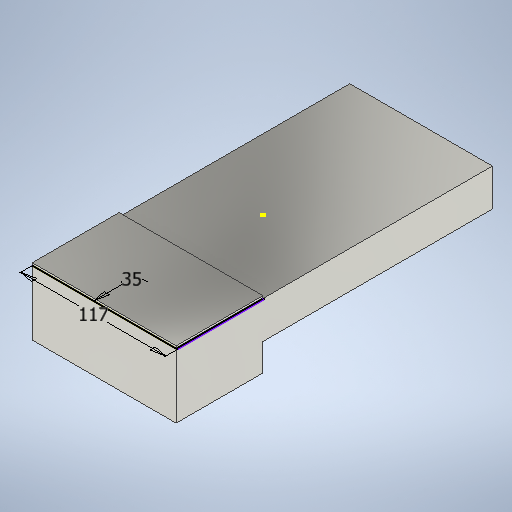
# Autodesk Inventor part: PSU
Saved by Autodesk Inventor 2025.1 (Build 291241000, 241)
## iProperties
Created: 2025-02-21
Part Number: PSU
Material: Generic
Document SubType Name: Modeling
Designer: m_kni
Density: 1 g/cm^3
Appearance: Default
Author: m_kni
Autodesk Inventor part; units mm, degrees
ref_plane "YZ Plane" through (0, 0, 0) normal (1, 0, 0) x (0, 1, 0)
ref_plane "XZ Plane" through (0, 0, 0) normal (0, 1, 0) x (-1, 0, 0)
ref_plane "XY Plane" through (0, 0, 0) normal (0, 0, 1) x (1, 0, 0)
sketch "Sketch1" plane through (0, 0, 0) normal (0, 1, 0) x (-1, 0, 0)
  line L0 (-57.5, -127.5) -> (57.5, -127.5)
  line L1 (57.5, -127.5) -> (57.5, 127.5)
  line L2 (57.5, 127.5) -> (-57.5, 127.5)
  line L3 (-57.5, 127.5) -> (-57.5, -127.5)
  line L4 (-57.5, -127.5) -> (57.5, 127.5) construction
  line L5 (57.5, -127.5) -> (-57.5, 127.5) construction
  point P0 (0, 0)
  dimension "d0" = 115
  dimension "d1" = 255
  constraints: 12 end point, 2 midpoint, 2 parallel, 1 horizontal, 1 perpendicular
  measures "d0" distance of L2.end L1.end
  measures "d1" distance of L1.end L0.end
extrude "Extrusion1" add sketch "Sketch1" along normal blind 30
sketch "Sketch2" plane through (0, 30, 0) normal (0, 1, 0) x (1, 0, 0)
  line L0 (-57.5, -127.5) -> (57.5, -127.5) projected
  line L1 (58.5, -57.5) -> (-58.5, -57.5)
  line L2 (-58.5, -57.5) -> (-58.5, -127.5)
  line L3 (-58.5, -127.5) -> (58.5, -127.5)
  line L4 (58.5, -127.5) -> (58.5, -57.5)
  line L5 (58.5, -57.5) -> (-58.5, -127.5) construction
  line L6 (-58.5, -57.5) -> (58.5, -127.5) construction
  line L7 (57.5, -57.5) -> (57.5, -127.5)
  point P0 (0, 0)
  point P1 (0, -92.5)
  dimension "d4" = 35
  dimension "d5" = 117
  constraints: 14 end point, 2 midpoint, 2 parallel, 2 perpendicular, 2 point on line, 1 horizontal
  measures "d4" distance from line of point (0, -92.5) L0
  measures "d5" distance of L3.end L2.end
extrude "Extrusion2" add sketch "Sketch2" along normal blind 2 contours L3 L2 L1 L7 L0
extrude "Extrusion3" add sketch "Sketch2" against normal blind 52 contours L3 L2 L1 L7 L0
body "Solid1"
